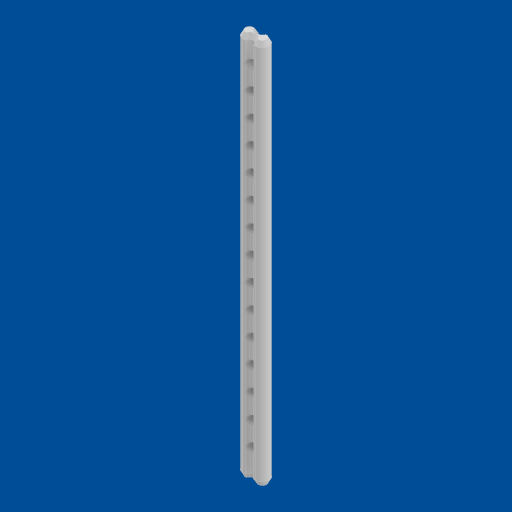
# Autodesk Inventor part: palca 325mm
Saved by Autodesk Inventor 2023 (Build 270158000, 158)
## iProperties
Created: 2021-11-23
Part Number: palca 325mm
Material: Generic
Document SubType Name: Modeling
Designer: Gábor
Density: 1 g/cm^3
Appearance: Default
Mass: 58.9549 g
Surface Area: 209.26 cm^2
Volume: 58.9549 cm^3
Author: Gábor
Autodesk Inventor part; units mm, degrees
ref_plane "YZ Plane" through (0, 0, 0) normal (1, 0, 0) x (0, 1, 0)
ref_plane "XZ Plane" through (0, 0, 0) normal (0, 1, 0) x (-1, 0, 0)
ref_plane "XY Plane" through (0, 0, 0) normal (0, 0, 1) x (1, 0, 0)
sketch "Sketch1" plane through (0, 0, 0) normal (0, 1, 0) x (-1, 0, 0)
  circle A0 centre (0, 0) radius 5.5
  circle A1 centre (-11, 0) radius 5.5
  circle A2 centre (0, 0) radius 7.5
  circle A3 centre (-11, 0) radius 7.5
  line L0 (0, 5.5) -> (-11, 5.5)
  line L1 (0, 0) -> (-3.5, 0)
  line L2 (-5.5, 0) -> (-5.5, 5.5)
  circle A4 centre (-5.5, 5.5) radius 3.25
  line L3 (0, -5.5) -> (-11, -5.5)
  circle A5 centre (-5.5, -5.5) radius 3.25
  point P0 (-8.75, 5.5)
  point P1 (-8.75, -5.5)
  point P2 (-2.25, -5.5)
  point P3 (-2.25, 5.5)
  dimension "d3" = 15
  dimension "d0" = 11
  dimension "d1" = 11
  dimension "d2" = 15
  dimension "d4" = 6.5
  constraints: 8 end point, 5 centre point, 4 coincident, 4 point on circle, 3 symmetric about line, 3 tangent, 1 horizontal, 1 horizontal alignment, 1 midpoint, 3 other
  measures "d0" diameter of A0
  measures "d1" diameter of A1
  measures "d2" diameter of A2
  measures "d4" diameter of A4
extrude "Extrusion1" add sketch "Sketch1" along normal blind 325 contours A0 A5 A3 A4 | A0 A4 L0 | L3 A5 A0 | A3 A5 A0 A4 | A0 L2 A4 | A5 A1 A0 | A1 A5 A2 A4 | A1 A4 L2 | A4 A1 L0 | L3 A1 A5 | A4 A2 A5 A1
chamfer "Chamfer1" distance 2 distance2 4 1 edges at (5.5, 325, -2.25) measured on face at (5.5, 325, -1.75)
chamfer "Chamfer2" distance 2 distance2 4 3 edges at (-5.5, 325, 0) (1.125, 325, 5.5) (0.125, 325, -5.5) measured on face at (-5, 325, 0) measured on face at (0.125, 325, -5.4) measured on face at (1.125, 325, 5)
chamfer "Chamfer3" distance 2 distance2 4 1 edges at (6.5576, 325, 2.4269) measured on face at (6.7203, 325, 1.9541)
chamfer "Chamfer4" distance 2 distance2 4 3 edges at (16.5, 325, 0) (10.875, 325, -5.5) (10.875, 325, 5.5) measured on face at (10.875, 325, 5.4) measured on face at (16, 325, 0) measured on face at (10.875, 325, -5.4)
chamfer "Chamfer5" distance 2 distance2 4 3 edges at (16.5, 0, 0) (9.875, 0, -5.5) (9.875, 0, 5.5) measured on face at (9.875, 0, 5) measured on face at (9.875, 0, -5) measured on face at (16, 0, 0)
chamfer "Chamfer6" distance 4 distance2 2 1 edges at (4.4424, 0, 2.4269) measured on face at (4.4424, 0.5, 2.4269)
chamfer "Chamfer7" distance 4 distance2 2 3 edges at (-5.5, 0, 0) (0.125, 0, 5.5) (1.125, 0, -5.5) measured on face at (-5.5, 0.5, 0) measured on face at (0.125, 0.1, 5.5) measured on face at (1.125, 0.5, -5.5)
chamfer "Chamfer8" distance 4 distance2 2 1 edges at (5.5, 0, -2.25) measured on face at (5.5, 0.5, -2.25)
sketch "Sketch2" plane through (0, 0, 0) normal (0, 0, 1) x (1, 0, 0)
  line L0 (8.75, 4) -> (2.25, 4) projected
  line L1 (5.5, 4) -> (4.9756, 325)
  line L2 (10.3541, 325) -> (0.6459, 325) projected
  line L3 (5.5, 4) -> (5.4673, 24)
  line L4 (0, 4) -> (0, 321) projected
  circle A0 centre (5.4673, 24) radius 3.25
  circle A1 centre (5.4347, 43.9999) radius 3.25
  line L5 (5.4673, 24) -> (4.943, 345)
  circle A2 centre (5.402, 63.9999) radius 3.25
  line L6 (5.4347, 43.9999) -> (4.9103, 364.9999)
  circle A3 centre (5.3693, 83.9999) radius 3.25
  line L7 (5.402, 63.9999) -> (4.8776, 384.9999)
  circle A4 centre (5.3366, 103.9999) radius 3.25
  line L8 (5.3693, 83.9999) -> (4.845, 404.9999)
  circle A5 centre (5.304, 123.9998) radius 3.25
  line L9 (5.3366, 103.9999) -> (4.8123, 424.9999)
  circle A6 centre (5.2713, 143.9998) radius 3.25
  line L10 (5.304, 123.9998) -> (4.7796, 444.9998)
  circle A7 centre (5.2386, 163.9998) radius 3.25
  line L11 (5.2713, 143.9998) -> (4.7469, 464.9998)
  circle A8 centre (5.206, 183.9998) radius 3.25
  line L12 (5.2386, 163.9998) -> (4.7143, 484.9998)
  circle A9 centre (5.1733, 203.9997) radius 3.25
  line L13 (5.206, 183.9998) -> (4.6816, 504.9998)
  circle A10 centre (5.1406, 223.9997) radius 3.25
  line L14 (5.1733, 203.9997) -> (4.6489, 524.9997)
  circle A11 centre (5.108, 243.9997) radius 3.25
  line L15 (5.1406, 223.9997) -> (4.6163, 544.9997)
  circle A12 centre (5.0753, 263.9997) radius 3.25
  line L16 (5.108, 243.9997) -> (4.5836, 564.9997)
  circle A13 centre (5.0426, 283.9996) radius 3.25
  line L17 (5.0753, 263.9997) -> (4.5509, 584.9997)
  circle A14 centre (5.0099, 303.9996) radius 3.25
  line L18 (5.0426, 283.9996) -> (4.5182, 604.9996)
  point P0 (0, 0)
  dimension "d31" = 20
  dimension "d33" = 6.5
  dimension "d36" = 20
  constraints: 32 end point, 16 point on line, 15 centre point, 15 coincident, 1 collinear, 1 midpoint, 84 other
  measures "d31" distance of L1.start L3.end
  measures "d33" diameter of A0
  measures "d36" distance of A0.centre A1.centre
extrude "Extrusion2" cut sketch "Sketch2" along normal mid plane 20
body "Solid1"
